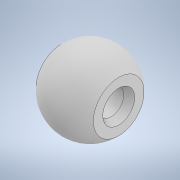
# Autodesk Inventor part: esfera
Saved by Autodesk Inventor 2022 (Build 260153000, 153)
## iProperties
Created: 2022-03-09
Part Number: esfera
Material: Generic
Document SubType Name: Modeling
Designer: Korch
Density: 1 g/cm^3
Appearance: Default
Author: Korch
Autodesk Inventor part; units mm, degrees
ref_plane "YZ Plane" through (0, 0, 0) normal (1, 0, 0) x (0, 1, 0)
ref_plane "XZ Plane" through (0, 0, 0) normal (0, 1, 0) x (-1, 0, 0)
ref_plane "XY Plane" through (0, 0, 0) normal (0, 0, 1) x (1, 0, 0)
sketch "Sketch1" plane through (0, 0, 0) normal (0, 0, 1) x (1, 0, 0)
  arc A0 (-4.5, -3.9686) -> (4.5, -3.9686) centre (0, 0) ccw
  arc A1 (4.5, 3.9686) -> (-4.5, 3.9686) centre (0, 0) ccw
  line L0 (-4.5, 0) -> (-4.5, 3.9686)
  line L1 (-4.5, 0) -> (-4.5, -3.9686)
  line L2 (4.5, 0) -> (4.5, 3.9686)
  line L3 (4.5, 0) -> (4.5, -3.9686)
  arc A2 (-4.5, -3.9686) -> (4.5, -3.9686) centre (0, 0) ccw
  arc A3 (4.5, 3.9686) -> (-4.5, 3.9686) centre (0, 0) ccw
  line L4 (-4.5, 0) -> (4.5, 0)
  constraints: 10 end point, 8 point on circle, 4 centre point, 3 vertical, 2 coincident, 1 perpendicular
revolve "Revolution1" [suppressed]
revolve "Revolution3" add sketch "Sketch1" angle 360 about axis through (-4.5, 0, 0) along (1, 0, 0) contours L0 A1 L2 L4
sketch "Sketch3" plane through (4.5, 0, 0) normal (1, 0, 0) x (0, 0, -1)
  point P0 (0, 0)
  point P1 (0, 0)
  constraints: 1 coincident
hole "Hole2" at (4.5, 0, 0) direction (-1, 0, 0) diameter 4 end through all countersink diameter 5 countersink angle 45
body "Solid1"
